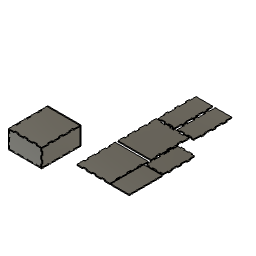
Locker_v2 (Autodesk Fusion 360 design; units mm, degrees)
Autodesk Fusion 360 part; units mm, degrees
sketch "Esquisse1" plane through (0, 0, 0) normal (0, 0, 1) x (1, 0, 0) in component "Base"
  line L0 (135, -160) -> (-135, -160)
  line L1 (-135, -160) -> (-135, 160)
  line L2 (-135, 160) -> (135, 160)
  line L3 (135, 160) -> (135, -160)
  line L4 (135, -160) -> (-135, 160) construction
  line L5 (-135, -160) -> (135, 160) construction
  line L6 (-90, 160) -> (-60, 160)
  line L7 (-60, 160) -> (-60, 151.8)
  line L8 (-60, 151.8) -> (-90, 151.8)
  line L9 (-90, 151.8) -> (-90, 160)
  line L10 (-15, 160) -> (15, 160)
  line L11 (15, 160) -> (15, 151.8)
  line L12 (15, 151.8) -> (-15, 151.8)
  line L13 (-15, 151.8) -> (-15, 160)
  line L14 (60, 160) -> (90, 160)
  line L15 (90, 160) -> (90, 151.8)
  line L16 (90, 151.8) -> (60, 151.8)
  line L17 (60, 151.8) -> (60, 160)
  line L18 (-90, 155.9) -> (-135, 155.9) construction
  line L19 (-60, 155.9) -> (-15, 155.9) construction
  line L20 (15, 155.9) -> (60, 155.9) construction
  line L21 (90, 155.9) -> (135, 155.9) construction
  line L22 (20, 0) -> (2.5, 0)
  line L23 (-90, -151.8) -> (-90, -160)
  line L24 (-60, -151.8) -> (-90, -151.8)
  line L25 (-60, -160) -> (-60, -151.8)
  line L26 (15, -151.8) -> (-15, -151.8)
  line L27 (-15, -151.8) -> (-15, -160)
  line L28 (15, -160) -> (15, -151.8)
  line L29 (90, -151.8) -> (60, -151.8)
  line L30 (90, -160) -> (90, -151.8)
  line L31 (60, -151.8) -> (60, -160)
  line L32 (135, 102.5) -> (126.8, 102.5)
  line L33 (126.8, 102.5) -> (126.8, 72.5)
  line L34 (126.8, 72.5) -> (135, 72.5)
  line L35 (135, 72.5) -> (135, 102.5)
  line L36 (135, 15) -> (126.8, 15)
  line L37 (126.8, 15) -> (126.8, -15)
  line L38 (126.8, -15) -> (135, -15)
  line L39 (135, -15) -> (135, 15)
  line L40 (135, -72.5) -> (126.8, -72.5)
  line L41 (126.8, -72.5) -> (126.8, -102.5)
  line L42 (126.8, -102.5) -> (135, -102.5)
  line L43 (135, -102.5) -> (135, -72.5)
  line L44 (130.9, 102.5) -> (130.9, 160) construction
  line L45 (130.9, 72.5) -> (130.9, 15) construction
  line L46 (130.9, -15) -> (130.9, -72.5) construction
  line L47 (130.9, -102.5) -> (130.9, -160) construction
  line L48 (0, 2.5) -> (0, 20)
  line L49 (-126.8, 102.5) -> (-126.8, 72.5)
  line L50 (-135, 102.5) -> (-126.8, 102.5)
  line L51 (-126.8, 72.5) -> (-135, 72.5)
  line L52 (-135, 15) -> (-126.8, 15)
  line L53 (-126.8, 15) -> (-126.8, -15)
  line L54 (-126.8, -15) -> (-135, -15)
  line L55 (-135, -72.5) -> (-126.8, -72.5)
  line L56 (-126.8, -72.5) -> (-126.8, -102.5)
  line L57 (-126.8, -102.5) -> (-135, -102.5)
  dimension "d6" = 270
  dimension "d7" = 320
  dimension "d8" = 8.2
  dimension "d9" = 30
  dimension "d10" = 30
  dimension "d11" = 8.2
  constraint horizontal L0
  constraint perpendicular L0 L1
  constraint parallel L0 L2
  constraint parallel L1 L3
  constraint coincident L4 origin
  constraint coincident L5 origin
  constraint horizontal L6
  constraint vertical L7
  constraint horizontal L8
  constraint vertical L9
  constraint coincident L2 L6.start
  constraint horizontal L10
  constraint vertical L11
  constraint horizontal L12
  constraint vertical L13
  constraint coincident L2 L10.start
  constraint horizontal L14
  constraint vertical L15
  constraint horizontal L16
  constraint vertical L17
  constraint coincident L2 L14.start
  constraint midpoint L9 L18.start
  constraint coincident L1 L18.end
  constraint perpendicular L1 L18
  constraint midpoint L7 L19.start
  constraint midpoint L13 L19.end
  constraint perpendicular L13 L19
  constraint midpoint L11 L20.start
  constraint midpoint L17 L20.end
  constraint perpendicular L17 L20
  constraint midpoint L15 L21.start
  constraint coincident L3 L21.end
  constraint perpendicular L3 L21
  constraint equal L19 L20
  constraint equal L18 L19
  constraint equal L18 L21
  constraint equal L8 L12
  constraint equal L12 L16
  constraint symmetric L6.start L22 L23.end
  constraint symmetric L6.end L22 L25.start
  constraint symmetric L7.end L22 L24.start
  constraint symmetric L8.end L22 L23.start
  constraint symmetric L10.start L22 L27.end
  constraint symmetric L10.end L22 L28.start
  constraint symmetric L11.end L22 L26.start
  constraint symmetric L12.end L22 L26.end
  constraint symmetric L14.start L22 L31.end
  constraint symmetric L14.end L22 L30.start
  constraint symmetric L15.end L22 L29.start
  constraint symmetric L16.end L22 L29.end
  constraint horizontal L32
  constraint vertical L33
  constraint horizontal L34
  constraint vertical L35
  constraint coincident L3 L32.start
  constraint horizontal L36
  constraint vertical L37
  constraint horizontal L38
  constraint vertical L39
  constraint coincident L3 L36.start
  constraint horizontal L40
  constraint vertical L41
  constraint horizontal L42
  constraint vertical L43
  constraint coincident L3 L40.start
  constraint midpoint L32 L44.start
  constraint coincident L2 L44.end
  constraint perpendicular L2 L44
  constraint midpoint L34 L45.start
  constraint midpoint L36 L45.end
  constraint perpendicular L36 L45
  constraint midpoint L38 L46.start
  constraint midpoint L40 L46.end
  constraint perpendicular L40 L46
  constraint midpoint L42 L47.start
  constraint coincident L0 L47.end
  constraint perpendicular L0 L47
  constraint equal L46 L47
  constraint equal L45 L46
  constraint equal L44 L45
  constraint equal L33 L37
  constraint equal L37 L41
  constraint symmetric L32.start L48 L50.start
  constraint symmetric L32.end L48 L49.start
  constraint symmetric L33.end L48 L49.end
  constraint symmetric L34.end L48 L51.end
  constraint symmetric L36.start L48 L52.start
  constraint symmetric L36.end L48 L52.end
  constraint symmetric L37.end L48 L53.end
  constraint symmetric L38.end L48 L54.end
  constraint symmetric L40.start L48 L55.start
  constraint symmetric L40.end L48 L55.end
  constraint symmetric L41.end L48 L56.end
  constraint symmetric L42.end L48 L57.end
  measures "d6" distance of L1.end L2.end
  measures "d7" distance of L0.end L1.end
  measures "d8" distance of L2 L12
  measures "d9" distance of L7.end L8.end
  measures "d10" distance of L32.end L33.end
  measures "d11" distance of L32.start L32.end
extrude "Extrusion1" add sketch "Esquisse1" along normal blind 8.2 contours L0 L1 L2 L3 L7 L8 L9 L11 L12 L13 L15 L16 L17 L23 L24 L25 L26 L27 L28 L29 L30 L31 L32 L33 L34 L36 L37 L38 L40 L41 L42 L49 L50 L51 L52 L53 L54 L55 L56 L57 makes body 1 in component "Base"
sketch "Esquisse1 (2)" plane through (135, 0, 0) normal (1, 0, 0) x (0, 1, 0) in component "long side"
  line L0 (-72.5, 0) -> (-15, 0)
  line L1 (-15, 0) -> (-15, 8.2)
  line L2 (-15, 8.2) -> (-72.5, 8.2)
  line L3 (-72.5, 8.2) -> (-72.5, 0)
  line L4 (-160, 0) -> (-102.5, 0)
  line L5 (-102.5, 0) -> (-102.5, 8.2)
  line L6 (-102.5, 8.2) -> (-160, 8.2)
  line L7 (-160, 8.2) -> (-160, 0)
  line L8 (-102.5, 0) -> (-72.5, 0)
  line L9 (-72.5, 0) -> (-72.5, 8.2)
  line L10 (-72.5, 8.2) -> (-102.5, 8.2)
  line L11 (-102.5, 8.2) -> (-102.5, 0)
  line L12 (-15, 0) -> (15, 0)
  line L13 (15, 0) -> (15, 8.2)
  line L14 (15, 8.2) -> (-15, 8.2)
  line L15 (-15, 8.2) -> (-15, 0)
  line L16 (15, 0) -> (72.5, 0)
  line L17 (72.5, 0) -> (72.5, 8.2)
  line L18 (72.5, 8.2) -> (15, 8.2)
  line L19 (15, 8.2) -> (15, 0)
  line L20 (72.5, 0) -> (102.5, 0)
  line L21 (102.5, 0) -> (102.5, 8.2)
  line L22 (102.5, 8.2) -> (72.5, 8.2)
  line L23 (72.5, 8.2) -> (72.5, 0)
  line L24 (102.5, 0) -> (160, 0)
  line L25 (160, 0) -> (160, 8.2)
  line L26 (160, 8.2) -> (102.5, 8.2)
  line L27 (102.5, 8.2) -> (102.5, 0)
  line L28 (-160, 0) -> (160, 0)
  line L29 (160, 0) -> (160, 150)
  line L30 (160, 150) -> (-160, 150)
  line L31 (-160, 150) -> (-160, 0)
  line L32 (-160, 120) -> (-151.8, 120)
  line L33 (-151.8, 120) -> (-151.8, 90)
  line L34 (-151.8, 90) -> (-160, 90)
  line L35 (-160, 90) -> (-160, 120)
  line L36 (-160, 60) -> (-151.8, 60)
  line L37 (-151.8, 60) -> (-151.8, 30)
  line L38 (-151.8, 30) -> (-160, 30)
  line L39 (-160, 30) -> (-160, 60)
  line L40 (-155.9, 120) -> (-155.9, 150) construction
  line L41 (-155.9, 90) -> (-155.9, 60) construction
  line L42 (-155.9, 30) -> (-155.9, 0) construction
  line L43 (0, 2.5) -> (0, 20)
  line L44 (160, 120) -> (151.8, 120)
  line L45 (151.8, 120) -> (151.8, 90)
  line L46 (151.8, 90) -> (160, 90)
  line L47 (160, 60) -> (151.8, 60)
  line L48 (151.8, 60) -> (151.8, 30)
  line L49 (151.8, 30) -> (160, 30)
  dimension "d14" = 150
  dimension "d15" = 8.2
  dimension "d16" = 30
  constraint horizontal L28
  constraint vertical L29
  constraint horizontal L30
  constraint vertical L31
  constraint coincident L4.start L7.end
  constraint coincident L25.end L29
  constraint horizontal L32
  constraint vertical L33
  constraint horizontal L34
  constraint vertical L35
  constraint coincident L31 L32.start
  constraint horizontal L36
  constraint vertical L37
  constraint horizontal L38
  constraint vertical L39
  constraint coincident L31 L36.start
  constraint midpoint L32 L40.start
  constraint coincident L30 L40.end
  constraint perpendicular L30 L40
  constraint midpoint L34 L41.start
  constraint midpoint L36 L41.end
  constraint perpendicular L36 L41
  constraint midpoint L38 L42.start
  constraint coincident L4 L42.end
  constraint equal L40 L41
  constraint equal L41 L42
  constraint vertical L42
  constraint equal L33 L37
  constraint symmetric L32.start L43 L44.start
  constraint symmetric L32.end L43 L44.end
  constraint symmetric L33.end L43 L45.end
  constraint symmetric L34.end L43 L46.end
  constraint symmetric L36.start L43 L47.start
  constraint symmetric L36.end L43 L47.end
  constraint symmetric L37.end L43 L48.end
  constraint symmetric L38.end L43 L49.end
  measures "d14" distance of L4.start L30.end
  measures "d15" distance of L37.end L38.end
  measures "d16" distance of L32.end L33.end
extrude "Extrusion1'" add sketch "Esquisse1 (2)" against normal blind 8.2 separate body contours L3 L5 L8 L9 L10 L11 L28 | L1 L12 L13 L14 L15 L19 L28 | L2 L6 L10 L14 L18 L22 L26 L29 L30 L31 L32 L33 L34 L36 L37 L38 L44 L45 L46 L47 L48 L49 | L17 L20 L21 L22 L23 L27 L28 makes body 2 in component "long side"
mirror "MirrorComponent1" about plane through (0, 0, 0) normal (0, 0, 1) of bodies 2 makes body 3 in component "long side(Symétrie miroir)"
sketch "Esquisse1 (3)" plane through (0, -160, 0) normal (0, -1, 0) x (1, 0, 0) in component "short side"
  line L0 (-135, 150) -> (-135, 120)
  line L1 (-135, 120) -> (-126.8, 120)
  line L2 (-126.8, 120) -> (-126.8, 150)
  line L3 (-126.8, 150) -> (-135, 150)
  line L4 (135, 8.2) -> (135, 30)
  line L5 (135, 30) -> (126.8, 30)
  line L6 (126.8, 30) -> (126.8, 8.2)
  line L7 (126.8, 8.2) -> (135, 8.2)
  line L8 (90, 0) -> (135, 0)
  line L9 (135, 0) -> (135, 8.2)
  line L10 (135, 8.2) -> (90, 8.2)
  line L11 (90, 8.2) -> (90, 0)
  line L12 (-135, 150) -> (135, 150)
  line L13 (135, 150) -> (135, 0)
  line L14 (135, 0) -> (-135, 0)
  line L15 (-135, 0) -> (-135, 150)
  constraint horizontal L12
  constraint vertical L13
  constraint horizontal L14
  constraint vertical L15
  constraint coincident L8.end L9.start
  constraint coincident L0.start L3.end
extrude "Extrusion1''" add sketch "Esquisse1 (3)" against normal blind 8.2 separate body makes body 4 in component "short side"
combine "Combiner1" operation cut target body 4 tool bodies 3 1 body 3 seen with x (-1, 0, 0) y (0, 1, 0) z (0, 0, -1) at (0, 0, 0) keep tools in component "short side"
mirror "MirrorComponent2" about plane through (0, 0, 0) normal (0, 0, 1) of bodies 4 makes body 5 in component "short side(Symétrie miroir)"
combine "Combiner2" operation cut target body 4 tool bodies 2 keep tools in component "short side"
combine "Combiner1'" operation cut target body 5 tool bodies 2 body 2 seen with x (1, 0, 0) y (0, -1, 0) z (0, 0, -1) at (0, 0, 0) keep tools in component "short side(Symétrie miroir)"
sketch "Esquisse1 (4)" plane through (0, 0, 150) normal (0, 0, 1) x (-1, 0, 0) in component "top"
  line L0 (-126.8, -151.8) -> (-126.8, -160)
  line L1 (-126.8, -160) -> (126.8, -160)
  line L2 (126.8, -160) -> (126.8, -151.8)
  line L3 (126.8, -151.8) -> (-126.8, -151.8)
  line L4 (135, 72.5) -> (126.8, 72.5)
  line L5 (126.8, 72.5) -> (126.8, 102.5)
  line L6 (126.8, 102.5) -> (135, 102.5)
  line L7 (135, 102.5) -> (135, 160)
  line L8 (135, 160) -> (90, 160)
  line L9 (90, 160) -> (90, 151.8)
  line L10 (90, 151.8) -> (60, 151.8)
  line L11 (60, 151.8) -> (60, 160)
  line L12 (60, 160) -> (15, 160)
  line L13 (15, 160) -> (15, 151.8)
  line L14 (15, 151.8) -> (-15, 151.8)
  line L15 (-15, 151.8) -> (-15, 160)
  line L16 (-15, 160) -> (-60, 160)
  line L17 (-60, 160) -> (-60, 151.8)
  line L18 (-60, 151.8) -> (-90, 151.8)
  line L19 (-90, 151.8) -> (-90, 160)
  line L20 (-90, 160) -> (-135, 160)
  line L21 (-135, 160) -> (-135, 102.5)
  line L22 (-135, 102.5) -> (-126.8, 102.5)
  line L23 (-126.8, 102.5) -> (-126.8, 72.5)
  line L24 (-126.8, 72.5) -> (-135, 72.5)
  line L25 (-135, 72.5) -> (-135, 15)
  line L26 (-135, 15) -> (-126.8, 15)
  line L27 (-126.8, 15) -> (-126.8, -15)
  line L28 (-126.8, -15) -> (-135, -15)
  line L29 (-135, -15) -> (-135, -72.5)
  line L30 (-135, -72.5) -> (-126.8, -72.5)
  line L31 (-126.8, -72.5) -> (-126.8, -102.5)
  line L32 (-126.8, -102.5) -> (-135, -102.5)
  line L33 (-135, -102.5) -> (-135, -160)
  line L34 (-135, -160) -> (-90, -160)
  line L35 (-90, -160) -> (-90, -151.8)
  line L36 (-90, -151.8) -> (-60, -151.8)
  line L37 (-60, -151.8) -> (-60, -160)
  line L38 (-60, -160) -> (-15, -160)
  line L39 (-15, -160) -> (-15, -151.8)
  line L40 (-15, -151.8) -> (15, -151.8)
  line L41 (15, -151.8) -> (15, -160)
  line L42 (15, -160) -> (60, -160)
  line L43 (60, -160) -> (60, -151.8)
  line L44 (60, -151.8) -> (90, -151.8)
  line L45 (90, -151.8) -> (90, -160)
  line L46 (90, -160) -> (135, -160)
  line L47 (135, -160) -> (135, -102.5)
  line L48 (135, -102.5) -> (126.8, -102.5)
  line L49 (126.8, -102.5) -> (126.8, -72.5)
  line L50 (126.8, -72.5) -> (135, -72.5)
  line L51 (135, -72.5) -> (135, -15)
  line L52 (135, -15) -> (126.8, -15)
  line L53 (126.8, -15) -> (126.8, 15)
  line L54 (126.8, 15) -> (135, 15)
  line L55 (135, 15) -> (135, 72.5)
extrude "Extrusion1'''" add sketch "Esquisse1 (4)" against normal blind 8.2 separate body contours L0 L1 L3 L34 L35 | L0 L2 L3 L4 L5 L6 L7 L8 L9 L10 L11 L12 L13 L14 L15 L16 L17 L18 L19 L20 L21 L22 L23 L24 L25 L26 L27 L28 L29 L30 L31 L32 L33 L34 L36 L40 L44 L46 L47 L48 L49 L50 L51 L52 L53 L54 L55 | L1 L3 L37 L38 L39 | L1 L3 L41 L42 L43 | L1 L2 L3 L45 L46 makes body 6 in component "top"
combine "Combiner1''" operation cut target body 3 tool bodies 6 body 6 seen with x (-1, 0, 0) y (0, 1, 0) z (0, 0, -1) at (0, 0, 0) keep tools in component "long side(Symétrie miroir)"
combine "Combiner2'" operation cut target body 5 tool bodies 6 body 6 seen with x (1, 0, 0) y (0, -1, 0) z (0, 0, -1) at (0, 0, 0) keep tools in component "short side(Symétrie miroir)"
combine "Combiner1'''" operation cut target body 2 tool bodies 6 keep tools in component "long side"
combine "Combiner3" operation cut target body 4 tool bodies 6 keep tools in component "short side"
sketch "Esquisse1 (5)" plane through (0, 160, 0) normal (0, 1, 0) x (-1, 0, 0) in component "Door"
  line L0 (-90, 150) -> (-135, 150)
  line L1 (-135, 150) -> (-135, 141.8)
  line L2 (-135, 141.8) -> (-90, 141.8)
  line L3 (-90, 141.8) -> (-90, 150)
  line L4 (-135, 150) -> (135, 150)
  line L5 (135, 150) -> (135, 0)
  line L6 (135, 0) -> (-135, 0)
  line L7 (-135, 0) -> (-135, 150)
  point P0 (-135, 150)
  point P1 (135, 150)
  point P2 (-135, 0)
  point P3 (135, 0)
  constraint horizontal L4
  constraint vertical L5
  constraint horizontal L6
  constraint vertical L7
  constraint coincident P3 L5.end
  constraint coincident P0 L0.end
extrude "Extrusion1''''" add sketch "Esquisse1 (5)" against normal blind 8.2 separate body makes body 7 in component "Door"
combine "Combiner2''" operation cut target body 2 tool bodies 7 keep tools in component "long side"
combine "Combiner1''''" operation cut target body 6 tool bodies 7 keep tools in component "top"
combine "Combiner2'''" operation cut target body 3 tool bodies 7 body 7 seen with x (-1, 0, 0) y (0, 1, 0) z (0, 0, -1) at (0, 0, 0) keep tools in component "long side(Symétrie miroir)"
combine "Combiner1'''''" operation cut target body 1 tool bodies 7 keep tools in component "Base"
other "Réorganiser1"
component "Base" placed x (1, 0, 0) y (0, 1, 0) z (0, 0, 1) at (0, 0, 0)
component "long side" placed x (1, 0, 0) y (0, 1, 0) z (0, 0, 1) at (0, 0, 0)
component "short side" placed x (1, 0, 0) y (0, 1, 0) z (0, 0, 1) at (0, 0, 0)
component "top" placed x (1, 0, 0) y (0, 1, 0) z (0, 0, 1) at (0, 0, 0)
component "Door" placed x (1, 0, 0) y (0, 1, 0) z (0, 0, 1) at (0, 0, 0)
component "long side(Symétrie miroir)" placed x (-1, 0, 0) y (0, 1, 0) z (0, 0, -1) at (0, 0, 0)
component "Réorganiser1" placed x (1, 0, 0) y (0, 1, 0) z (0, 0, 1) at (0, 0, 0)
component "Enveloppe1(Qté: 1)" placed x (1, 0, 0) y (0, 1, 0) z (0, 0, 1) at (250, 0, 0) in component "Réorganiser1"
component "Base" placed x (-1, 0, 0) y (0, 1, 0) z (0, 0, -1) at (141.35, 166.35, 9.2) in component "Enveloppe1(Qté: 1)"
component "long side" placed x (0, 0, 1) y (0, 1, 0) z (-1, 0, 0) at (312.7, 819.05, -125.8) in component "Enveloppe1(Qté: 1)"
component "long side(Symétrie miroir)" placed x (0, 0, 1) y (0, 1, 0) z (-1, 0, 0) at (6.35, 819.05, -125.8) in component "Enveloppe1(Qté: 1)"
component "short side" placed x (0, 1, 0) y (0, 0, -1) z (-1, 0, 0) at (432.7, 417.7, -150.8) in component "Enveloppe1(Qté: 1)"
component "top" placed x (-1, 0, 0) y (0, -1, 0) z (0, 0, 1) at (141.35, 492.7, -140.8) in component "Enveloppe1(Qté: 1)"
component "Door" placed x (0, -1, 0) y (0, 0, 1) z (-1, 0, 0) at (432.7, 141.35, -150.8) in component "Enveloppe1(Qté: 1)"
equation "depth = 320 mm"
equation "width = 270 mm"
equation "ply = 8.2 mm"
equation "holeSpace = depth / 5"
equation "height = 150 mm"
equation "d6 = width"
equation "d7 = depth"
equation "d8 = ply"
equation "d9 = tab"
equation "d10 = d9"
equation "d11 = ply"
equation "d12 = ply"
equation "d14 = height"
equation "d15 = ply"
equation "d16 = tab"
equation "d17 = -ply"
equation "d19 = -ply"
equation "tab = 30 mm"
equation "d22 = -ply"
equation "d24 = -ply"
